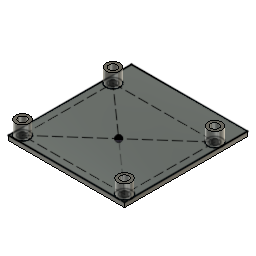
BTT24V_UPS_Module (Autodesk Fusion 360 design; units mm, degrees)
Autodesk Fusion 360 part; units mm, degrees
sketch "Sketch1" plane through (0, 0, 0) normal (0, 0, 1) x (1, 0, 0)
  line L0 (25, -22.5) -> (-25, -22.5)
  line L1 (-25, -22.5) -> (-25, 30.5)
  line L2 (-25, 30.5) -> (25, 30.5)
  line L3 (25, 30.5) -> (25, -22.5)
  line L4 (22, -19.5) -> (-22, -19.5) construction
  line L5 (-22, -19.5) -> (-22, 19.5) construction
  line L6 (-22, 19.5) -> (22, 19.5) construction
  line L7 (22, 19.5) -> (22, -19.5) construction
  line L8 (22, -19.5) -> (-22, 19.5) construction
  line L9 (-22, -19.5) -> (22, 19.5) construction
  circle A0 centre (-22, 19.5) radius 1.75
  circle A1 centre (22, 19.5) radius 1.75
  circle A2 centre (22, -19.5) radius 1.75
  circle A3 centre (-22, -19.5) radius 1.75
  circle A4 centre (-22, -19.5) radius 3
  circle A5 centre (-22, 19.5) radius 3
  circle A6 centre (22, 19.5) radius 3
  circle A7 centre (22, -19.5) radius 3
  dimension "d1" = 50
  dimension "d2" = 53
  dimension "d3" = 39
  dimension "d4" = 44
  dimension "d5" = 3
  dimension "d6" = 3
  dimension "d7" = 3.5
  dimension "d8" = 3.5
  dimension "d9" = 3.5
  dimension "d10" = 3.5
  dimension "d11" = 6
  dimension "d12" = 6
  dimension "d13" = 6
  dimension "d14" = 6
  constraint perpendicular L0 L1
  constraint parallel L0 L2
  constraint parallel L1 L3
  constraint horizontal L0
  constraint perpendicular L4 L5
  constraint parallel L4 L6
  constraint parallel L5 L7
  constraint horizontal L4
  constraint coincident L8 origin
  constraint coincident L9 origin
  constraint coincident L5.end L6.start
  constraint coincident L6.end L7.start
  constraint coincident L4.start L7.end
  constraint coincident L4.end L5.start
  constraint concentric A3 A4
  constraint concentric A0 A5
  constraint concentric A1 A6
  constraint concentric A2 A7
  measures "d1" distance of L1.end L2.end
  measures "d2" distance of L0.end L1.end
  measures "d3" distance of L4.end L5.end
  measures "d4" distance of L5.end L6.end
  measures "d5" distance of L3 L7
  measures "d6" distance of L0 L4
  measures "d7" diameter of A0
  measures "d8" diameter of A1
  measures "d9" diameter of A2
  measures "d10" diameter of A3
  measures "d11" diameter of A4 L0.start
  measures "d12" diameter of A5
  measures "d13" diameter of A6
  measures "d14" diameter of A7 L0.start
extrude "Extrude1" add sketch "Sketch1" against normal blind 2 contours L0 L3 A7 | A6 | A5 | L0 L1 L2 L3 A4 A7 | A7 | L0 L1 A4 | A4 | A0 | A1 | A2 | A3
extrude "Extrude2" add sketch "Sketch1" along normal blind 6 contours A6 | A5 | A7 | A4
